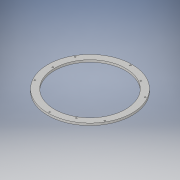
# Autodesk Inventor part: Slewing Bearing
Saved by Autodesk Inventor 2019.4 (Build 234330000, 330)
## iProperties
Created: 2020-01-19
Part Number: Slewing Bearing
Material: Aluminum 6061
Document SubType Name: Modeling
Designer: admin
Mass: 670 g
Surface Area: 740.328 cm^2
Volume: 244.656 cm^3
Density: 2.73854 g/cm^3
Appearance: Aluminum Cast
Author: admin
Autodesk Inventor part; units mm, degrees
ref_plane "YZ Plane" through (0, 0, 0) normal (1, 0, 0) x (0, 1, 0)
ref_plane "XZ Plane" through (0, 0, 0) normal (0, 1, 0) x (-1, 0, 0)
ref_plane "XY Plane" through (0, 0, 0) normal (0, 0, 1) x (1, 0, 0)
sketch "Sketch1" plane through (0, 0, 0) normal (0, 1, 0) x (-1, 0, 0)
  circle A0 centre (0, 0) radius 148
  circle A1 centre (0, 0) radius 175
  line L0 (154.7299, 0) -> (-77.3649, -134) construction
  line L1 (-77.3649, -134) -> (-77.3649, 134) construction
  line L2 (-77.3649, 134) -> (154.7299, 0) construction
  line L3 (145.7088, -84.125) -> (0, -168.25) construction
  line L4 (0, -168.25) -> (-145.7088, -84.125) construction
  line L5 (-145.7088, -84.125) -> (-145.7088, 84.125) construction
  line L6 (-145.7088, 84.125) -> (0, 168.25) construction
  line L7 (0, 168.25) -> (145.7088, 84.125) construction
  line L8 (145.7088, 84.125) -> (145.7088, -84.125) construction
  circle A2 centre (-145.7088, 84.125) radius 2.75
  circle A3 centre (-145.7088, -84.125) radius 2.75
  circle A4 centre (-77.3649, -134) radius 2.75
  circle A5 centre (0, -168.25) radius 2.75
  circle A6 centre (145.7088, -84.125) radius 2.75
  circle A7 centre (154.7299, 0) radius 2.75
  circle A8 centre (145.7088, 84.125) radius 2.75
  circle A9 centre (0, 168.25) radius 2.75
  circle A10 centre (-77.3649, 134) radius 2.75
  dimension "d0" = 296
  dimension "d1" = 350
  dimension "d2" = 268
  dimension "d3" = 336.5
  dimension "d4" = 5.5
  dimension "d5" = 5.5
  dimension "d6" = 5.5
  dimension "d7" = 5.5
  dimension "d8" = 5.5
  dimension "d9" = 5.5
  dimension "d10" = 5.5
  dimension "d11" = 5.5
  dimension "d12" = 5.5
  constraints: 18 end point, 13 coincident, 11 centre point, 2 vertical, 20 other
  measures "d0" diameter of A0
  measures "d1" diameter of A1
  measures "d2" distance of L0.end L1.end
  measures "d3" distance of L3.end L6.end
  measures "d4" diameter of A2
  measures "d5" diameter of A3
  measures "d6" diameter of A4
  measures "d7" diameter of A5
  measures "d8" diameter of A6
  measures "d9" diameter of A7
  measures "d10" diameter of A8
  measures "d11" diameter of A9
  measures "d12" diameter of A10
extrude "Extrusion1" add sketch "Sketch1" along normal blind 9
body "Solid1"
